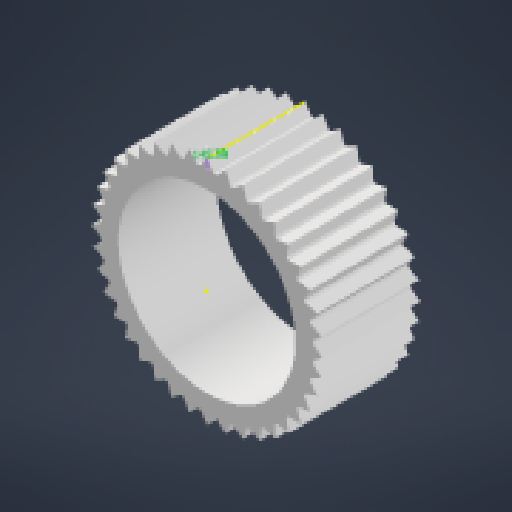
# Autodesk Inventor part: 60mm Wheel Tire Tread
Saved by Autodesk Inventor 2024 (Build 280153000, 153)
## iProperties
Created: 2023-09-10
Part Number: 60mm Wheel Tire Tread
Material: Generic
Document SubType Name: Modeling
Designer: izack
Density: 1 g/cm^3
Appearance: Default
Author: izack
Autodesk Inventor part; units mm, degrees
ref_plane "YZ Plane" through (0, 0, 0) normal (1, 0, 0) x (0, 1, 0)
ref_plane "XZ Plane" through (0, 0, 0) normal (0, 1, 0) x (-1, 0, 0)
ref_plane "XY Plane" through (0, 0, 0) normal (0, 0, 1) x (1, 0, 0)
sketch "Sketch1" plane through (0, 0, 0) normal (0, 0, 1) x (1, 0, 0)
  circle A0 centre (0, 0) radius 22.888 projected
  circle A1 centre (0, 0) radius 30
  dimension "d0" = 60
  constraints: 1 centre point, 1 coincident
  measures "d0" diameter of A1
extrude "Extrusion1" add sketch "Sketch1" against normal blind 25.4
sketch "Sketch2" plane through (0, 0, 0) normal (0, 0, 1) x (1, 0, 0)
  circle A0 centre (0, 0) radius 30 projected
  circle A1 centre (0, 0) radius 22.888 projected
  circle A2 centre (0, 0) radius 27.46
  line L0 (0, 27.46) -> (0, 30) construction
  line L1 (0, 30) -> (-1.8208, 27.3996)
  line L2 (0, 30) -> (1.8208, 27.3996)
  line L3 (0, 0) -> (0, 39.6281) construction
  line L4 (-4.693, 29.6307) -> (-6.0847, 26.7774)
  line L5 (-4.693, 29.6307) -> (-2.4878, 27.3471)
  line L6 (-9.2705, 28.5317) -> (-10.1987, 25.4959)
  line L7 (-9.2705, 28.5317) -> (-6.7352, 26.6212)
  line L8 (-13.6197, 26.7302) -> (-14.0615, 23.5865)
  line L9 (-13.6197, 26.7302) -> (-10.8168, 25.2398)
  line L10 (-17.6336, 24.2705) -> (-17.5782, 21.0964)
  line L11 (-17.6336, 24.2705) -> (-14.632, 23.237)
  line L12 (-21.2132, 21.2132) -> (-20.6619, 18.0869)
  line L13 (-21.2132, 21.2132) -> (-18.0869, 20.6619)
  line L14 (-24.2705, 17.6336) -> (-23.237, 14.632)
  line L15 (-24.2705, 17.6336) -> (-21.0964, 17.5782)
  line L16 (-26.7302, 13.6197) -> (-25.2398, 10.8168)
  line L17 (-26.7302, 13.6197) -> (-23.5865, 14.0615)
  line L18 (-28.5317, 9.2705) -> (-26.6212, 6.7352)
  line L19 (-28.5317, 9.2705) -> (-25.4959, 10.1987)
  line L20 (-29.6307, 4.693) -> (-27.3471, 2.4878)
  line L21 (-29.6307, 4.693) -> (-26.7774, 6.0847)
  line L22 (-30, 0) -> (-27.3996, -1.8208)
  line L23 (-30, 0) -> (-27.3996, 1.8208)
  line L24 (-29.6307, -4.693) -> (-26.7774, -6.0847)
  line L25 (-29.6307, -4.693) -> (-27.3471, -2.4878)
  line L26 (-28.5317, -9.2705) -> (-25.4959, -10.1987)
  line L27 (-28.5317, -9.2705) -> (-26.6212, -6.7352)
  line L28 (-26.7302, -13.6197) -> (-23.5865, -14.0615)
  line L29 (-26.7302, -13.6197) -> (-25.2398, -10.8168)
  line L30 (-24.2705, -17.6336) -> (-21.0964, -17.5782)
  line L31 (-24.2705, -17.6336) -> (-23.237, -14.632)
  line L32 (-21.2132, -21.2132) -> (-18.0869, -20.6619)
  line L33 (-21.2132, -21.2132) -> (-20.6619, -18.0869)
  line L34 (-17.6336, -24.2705) -> (-14.632, -23.237)
  line L35 (-17.6336, -24.2705) -> (-17.5782, -21.0964)
  line L36 (-13.6197, -26.7302) -> (-10.8168, -25.2398)
  line L37 (-13.6197, -26.7302) -> (-14.0615, -23.5865)
  line L38 (-9.2705, -28.5317) -> (-6.7352, -26.6212)
  line L39 (-9.2705, -28.5317) -> (-10.1987, -25.4959)
  line L40 (-4.693, -29.6307) -> (-2.4878, -27.3471)
  line L41 (-4.693, -29.6307) -> (-6.0847, -26.7774)
  line L42 (0, -30) -> (1.8208, -27.3996)
  line L43 (0, -30) -> (-1.8208, -27.3996)
  line L44 (4.693, -29.6307) -> (6.0847, -26.7774)
  line L45 (4.693, -29.6307) -> (2.4878, -27.3471)
  line L46 (9.2705, -28.5317) -> (10.1987, -25.4959)
  line L47 (9.2705, -28.5317) -> (6.7352, -26.6212)
  line L48 (13.6197, -26.7302) -> (14.0615, -23.5865)
  line L49 (13.6197, -26.7302) -> (10.8168, -25.2398)
  line L50 (17.6336, -24.2705) -> (17.5782, -21.0964)
  line L51 (17.6336, -24.2705) -> (14.632, -23.237)
  line L52 (21.2132, -21.2132) -> (20.6619, -18.0869)
  line L53 (21.2132, -21.2132) -> (18.0869, -20.6619)
  line L54 (24.2705, -17.6336) -> (23.237, -14.632)
  line L55 (24.2705, -17.6336) -> (21.0964, -17.5782)
  line L56 (26.7302, -13.6197) -> (25.2398, -10.8168)
  line L57 (26.7302, -13.6197) -> (23.5865, -14.0615)
  line L58 (28.5317, -9.2705) -> (26.6212, -6.7352)
  line L59 (28.5317, -9.2705) -> (25.4959, -10.1987)
  line L60 (29.6307, -4.693) -> (27.3471, -2.4878)
  line L61 (29.6307, -4.693) -> (26.7774, -6.0847)
  line L62 (30, 0) -> (27.3996, 1.8208)
  line L63 (30, 0) -> (27.3996, -1.8208)
  line L64 (29.6307, 4.693) -> (26.7774, 6.0847)
  line L65 (29.6307, 4.693) -> (27.3471, 2.4878)
  line L66 (28.5317, 9.2705) -> (25.4959, 10.1987)
  line L67 (28.5317, 9.2705) -> (26.6212, 6.7352)
  line L68 (26.7302, 13.6197) -> (23.5865, 14.0615)
  line L69 (26.7302, 13.6197) -> (25.2398, 10.8168)
  line L70 (24.2705, 17.6336) -> (21.0964, 17.5782)
  line L71 (24.2705, 17.6336) -> (23.237, 14.632)
  line L72 (21.2132, 21.2132) -> (18.0869, 20.6619)
  line L73 (21.2132, 21.2132) -> (20.6619, 18.0869)
  line L74 (17.6336, 24.2705) -> (14.632, 23.237)
  line L75 (17.6336, 24.2705) -> (17.5782, 21.0964)
  line L76 (13.6197, 26.7302) -> (10.8168, 25.2398)
  line L77 (13.6197, 26.7302) -> (14.0615, 23.5865)
  line L78 (9.2705, 28.5317) -> (6.7352, 26.6212)
  line L79 (9.2705, 28.5317) -> (10.1987, 25.4959)
  line L80 (4.693, 29.6307) -> (2.4878, 27.3471)
  line L81 (4.693, 29.6307) -> (6.0847, 26.7774)
  point P0 (30, 0)
  point P1 (30, 0)
  dimension "d3" = 2.54
  dimension "d4" = 35
  dimension "d5" = 35
  dimension "d10" = 360
  constraints: 164 end point, 2 vertical, 1 collinear, 206 other
  measures "d4" angle of L0 L1
  measures "d5" angle of L0 L2
extrude "Extrusion2" cut sketch "Sketch2" against normal blind 25.4 contours L62 A2 L65 A0 | A0 L60 A2 L63 | L64 A2 L67 A0 | A0 L58 A2 L61 | L66 A2 L69 A0 | A0 L56 A2 L59 | L68 A2 L71 A0 | A0 L54 A2 L57 | L70 A2 L73 A0 | A0 L52 A2 L55 | L72 A2 L75 A0 | A0 L50 A2 L53 | L74 A2 L77 A0 | A0 L48 A2 L51 | L76 A2 L79 A0 | A0 L46 A2 L49 | L78 A2 L81 A0 | A0 L44 A2 L47 | L80 A2 L2 A0 | A0 L42 A2 L45 | L1 A2 L5 A0 | A0 L40 A2 L43 | L4 A2 L7 A0 | A0 L38 A2 L41 | L6 A2 L9 A0 | A0 L36 A2 L39 | L8 A2 L11 A0 | A0 L34 A2 L37 | L10 A2 L13 A0 | A0 L32 A2 L35 | L12 A2 L15 A0 | A0 L30 A2 L33 | L14 A2 L17 A0 | A0 L28 A2 L31 | L16 A2 L19 A0 | A0 L26 A2 L29 | L18 A2 L21 A0 | A0 L24 A2 L27 | L20 A2 L23 A0 | A0 L22 A2 L25
sketch "Sketch3" plane through (0, 0, 0) normal (1, 0, 0) x (0, 1, 0)
  line L0 (30, 0) -> (30, -25.4) projected
  line L1 (30, 0) -> (27.3996, 0) projected
  line L2 (27.3996, 0) -> (27.3996, -25.4) projected
  line L3 (30, 0) -> (27.3996, 0)
  line L4 (27.3996, 0) -> (27.3996, -25.4)
  line L5 (27.3996, -25.4) -> (30, -25.4)
  line L6 (30, 0) -> (27.3996, -1.8208)
  line L7 (30, 0) -> (33.1745, 0) construction
  line L8 (27.3996, -1.8208) -> (30, -1.8208) construction
  line L9 (30, -3.6417) -> (27.3996, -1.8208)
  line L10 (30, -4.318) -> (27.3996, -6.1388)
  line L11 (30, -7.9597) -> (27.3996, -6.1388)
  line L12 (30, -8.636) -> (27.3996, -10.4568)
  line L13 (30, -12.2777) -> (27.3996, -10.4568)
  line L14 (30, -12.954) -> (27.3996, -14.7748)
  line L15 (30, -16.5957) -> (27.3996, -14.7748)
  line L16 (30, -17.272) -> (27.3996, -19.0928)
  line L17 (30, -20.9137) -> (27.3996, -19.0928)
  line L18 (30, -21.59) -> (27.3996, -23.4108)
  line L19 (30, -25.2317) -> (27.3996, -23.4108)
  line L20 (0, 0) -> (0, -25.2317) construction
  dimension "d12" = 145
  dimension "d15" = 4.318
  constraints: 36 end point, 3 perpendicular, 2 point on line, 2 vertical, 1 collinear, 1 equal length, 1 horizontal, 1 symmetric about line, 25 other
  measures "d12" angle of L6 L7
  measures "d15" distance of L0.start L10.start
revolve "Revolution1" cut sketch "Sketch3" angle 360 about axis through (0, 0, 0) along (0, 0, -1) contours L0 L9 L6 | L0 L11 L10 | L12 L0 L13 | L14 L0 L15 | L16 L0 L17 | L18 L0 L19
body "Solid1"
